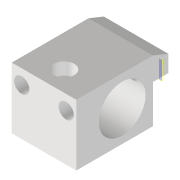
# Autodesk Inventor part: 40_XYZstage_micrometer_motorized_nema8_nanotec_adapter
Saved by Autodesk Inventor 2022 (Build 260153000, 153)
## iProperties
Created: 2023-04-17
Part Number: 40_XYZstage_micrometer_motorized_nema8_nanotec_adapter
Material: Generisch
Document SubType Name: Modeling
Designer: diederichbenedict
Density: 1 g/cm^3
Appearance: Vorgabe
Author: diederichbenedict
Autodesk Inventor part; units mm, degrees
ref_plane "YZ Plane" through (0, 0, 0) normal (1, 0, 0) x (0, 1, 0)
ref_plane "XZ Plane" through (0, 0, 0) normal (0, 1, 0) x (-1, 0, 0)
ref_plane "XY Plane" through (0, 0, 0) normal (0, 0, 1) x (1, 0, 0)
sketch "Skizze1" plane through (0, 0, 0) normal (0, 0, 1) x (1, 0, 0)
  line L0 (10.5, -2.75) -> (-10.5, -2.75)
  line L1 (-10.5, -2.75) -> (-10.5, 2.75)
  line L2 (-10.5, 2.75) -> (10.5, 2.75)
  line L3 (10.5, 2.75) -> (10.5, -2.75)
  line L4 (10.5, -2.75) -> (-10.5, 2.75) construction
  line L5 (-10.5, -2.75) -> (10.5, 2.75) construction
  circle A0 centre (7.25, 0) radius 1.25
  circle A1 centre (-7.25, 0) radius 1.25
  point P0 (0, 0)
  dimension "d0" = 21
  dimension "d1" = 5.5
  dimension "d2" = 2.5
  dimension "d3" = 2.5
  dimension "d4" = 7.25
  dimension "d5" = 7.25
  constraints: 12 end point, 2 centre point, 2 midpoint, 2 parallel, 1 horizontal, 1 perpendicular
  measures "d0" distance of L1.end L2.end
  measures "d1" distance of L0.end L1.end
  measures "d2" diameter of A0
  measures "d3" diameter of A1
  measures "d4" distance of A1.centre point (0, 0)
  measures "d5" distance of A0.centre point (0, 0)
extrude "Extrusion1" add sketch "Skizze1" along normal blind 5
sketch "Skizze2" plane through (0, 0, 0) normal (1, 0, 0) x (0, 1, 0)
  line L0 (-2.75, 0) -> (2.75, 0) projected
  line L1 (2.75, 0) -> (2.75, 5) projected
  line L2 (-2.75, 5) -> (2.75, 5) projected
  line L3 (-2.75, 0) -> (-2.75, 5) projected
  line L4 (4.75, 5) -> (-15.25, 5)
  line L5 (-15.25, 5) -> (-15.25, 30)
  line L6 (-15.25, 30) -> (4.75, 30)
  line L7 (4.75, 30) -> (4.75, 5)
  circle A0 centre (-5.25, 15) radius 7.25
  line L8 (2.75, 0) -> (4.75, 5)
  line L9 (-2.75, 0) -> (-15.25, 5)
  point P0 (0, 0)
  dimension "d8" = 20
  dimension "d9" = 25
  dimension "d10" = 2
  dimension "d11" = 14.5
  constraints: 12 end point, 2 parallel, 2 perpendicular, 1 centre point, 1 horizontal
  measures "d8" distance of L5.end L6.end
  measures "d9" distance of L4.end L5.end
  measures "d10" distance between parallel lines of L1 L7
  measures "d11" diameter of A0
extrude "Extrusion2" add sketch "Skizze2" along normal mid plane 21 contours L1 L4 L8 | L4 L5 L6 L7 L2
ref_plane "Arbeitsebene1" through (0, 0, 3) normal (0, 0, -1) x (-1, 0, 0)
sketch "Skizze3" plane through (0, 0, 3) normal (0, 0, -1) x (-1, 0, 0)
  circle A0 centre (7.25, 0) radius 1.25 projected
  circle A1 centre (-7.25, 0) radius 1.25 projected
  circle A2 centre (7.25, 0) radius 1.25 projected
  circle A3 centre (7.25, 0) radius 2.5
  circle A4 centre (-7.25, 0) radius 2.5
  point P0 (0, 0)
  dimension "d15" = 5
  dimension "d16" = 5
  constraints: 2 centre point, 2 coincident
  measures "d15" diameter of A3
  measures "d16" diameter of A4
extrude "Extrusion3" cut sketch "Skizze3" against normal through all contours A0 | A1 | A3 | A4
sketch "Skizze4" plane through (-10.5, 4.75, 30) normal (0, 1, 0) x (1, 0, 0)
  line L0 (21, 0) -> (0, 0) projected
  line L1 (21, 25) -> (21, 0) projected
  line L2 (0, 25) -> (21, 25) projected
  line L3 (0, 0) -> (0, 25) projected
  line L4 (21, 7.75) -> (0, 7.75) projected
  circle A0 centre (10.5, 6.5785) radius 1.4
  point P0 (10.5, 30)
  dimension "d19" = 2.8
  constraints: 1 centre point
  measures "d19" diameter of A0
hole "Bohrung1" at (0, 4.75, 23.4215) direction (0, -1, 0) diameter 2.8 end through all counterbore diameter 6.5 counterbore depth 4
sketch "Skizze5" plane through (-10.5, -2.75, 0) normal (-1, 0, 0) x (0, 0, 1)
  circle A0 centre (15, -2.5) radius 7.25 projected
  point P0 (0, 2.75)
extrude "Extrusion4" cut sketch "Skizze5" against normal through all draft 1
